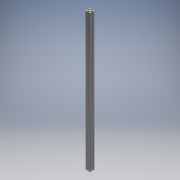
# Autodesk Inventor part: 4040_Alu
Saved by Autodesk Inventor 2019 (Build 230136000, 136)
## iProperties
Created: 2018-02-07
Part Number: 4040_Alu
Material: Aluminum 6061
Document SubType Name: Modeling
Designer: thijs
Density: 2.7 g/cm^3
Appearance: Aluminum - Polished
Author: thijs
Autodesk Inventor part; units mm, degrees
ref_plane "YZ Plane" through (0, 0, 0) normal (1, 0, 0) x (0, 1, 0)
ref_plane "XZ Plane" through (0, 0, 0) normal (0, 1, 0) x (-1, 0, 0)
ref_plane "XY Plane" through (0, 0, 0) normal (0, 0, 1) x (1, 0, 0)
sketch "Sketch1" plane through (0, 0, 0) normal (0, 0, 1) x (1, 0, 0)
  line L0 (7.425, -7.425) -> (-7.425, -7.425)
  line L1 (-7.425, -7.425) -> (-7.425, 7.425)
  line L2 (-7.425, 7.425) -> (7.425, 7.425)
  line L3 (7.425, 7.425) -> (7.425, -7.425)
  line L4 (7.425, -7.425) -> (-7.425, 7.425) construction
  line L5 (-7.425, -7.425) -> (7.425, 7.425) construction
  line L6 (20, -20) -> (-20, -20)
  line L7 (-20, -20) -> (-20, 20)
  line L8 (-20, 20) -> (20, 20)
  line L9 (20, 20) -> (20, -20)
  line L10 (20, -20) -> (-20, 20) construction
  line L11 (-20, -20) -> (20, 20) construction
  line L12 (-16.1503, -19.205) -> (19.205, 16.1503)
  line L13 (19.205, 16.1503) -> (16.1503, 19.205)
  line L14 (16.1503, 19.205) -> (-19.205, -16.1503)
  line L15 (-19.205, -16.1503) -> (-16.1503, -19.205)
  line L16 (-16.1503, -19.205) -> (16.1503, 19.205) construction
  line L17 (19.205, 16.1503) -> (-19.205, -16.1503) construction
  line L18 (16.1503, -19.205) -> (-19.205, 16.1503)
  line L19 (-19.205, 16.1503) -> (-16.1503, 19.205)
  line L20 (-16.1503, 19.205) -> (19.205, -16.1503)
  line L21 (19.205, -16.1503) -> (16.1503, -19.205)
  line L22 (16.1503, -19.205) -> (-16.1503, 19.205) construction
  line L23 (-19.205, 16.1503) -> (19.205, -16.1503) construction
  line L24 (-20, 20) -> (-15.68, 20)
  line L25 (-15.68, 20) -> (-15.68, 4.065)
  line L26 (-15.68, 4.065) -> (-20, 4.065)
  line L27 (-20, 4.065) -> (-20, 20)
  line L28 (-20, -20) -> (-15.68, -20)
  line L29 (-15.68, -20) -> (-15.68, -4.065)
  line L30 (-15.68, -4.065) -> (-20, -4.065)
  line L31 (-20, -4.065) -> (-20, -20)
  line L32 (-20, 20) -> (-4.32, 20)
  line L33 (-4.32, 20) -> (-4.32, 15.68)
  line L34 (-4.32, 15.68) -> (-20, 15.68)
  line L35 (-20, 15.68) -> (-20, 20)
  line L36 (20, 20) -> (3.81, 20)
  line L37 (3.81, 20) -> (3.81, 15.68)
  line L38 (3.81, 15.68) -> (20, 15.68)
  line L39 (20, 15.68) -> (20, 20)
  line L40 (20, -20) -> (15.68, -20)
  line L41 (15.68, -20) -> (15.68, -4.32)
  line L42 (15.68, -4.32) -> (20, -4.32)
  line L43 (20, -4.32) -> (20, -20)
  line L44 (20, -20) -> (4.065, -20)
  line L45 (4.065, -20) -> (4.065, -15.68)
  line L46 (4.065, -15.68) -> (20, -15.68)
  line L47 (20, -15.68) -> (20, -20)
  line L48 (-20, -20) -> (-4.065, -20)
  line L49 (-4.065, -20) -> (-4.065, -15.68)
  line L50 (-4.065, -15.68) -> (-20, -15.68)
  line L51 (-20, -15.68) -> (-20, -20)
  line L52 (20, 20) -> (15.68, 20)
  line L53 (15.68, 20) -> (15.68, 3.81)
  line L54 (15.68, 3.81) -> (20, 3.81)
  line L55 (20, 3.81) -> (20, 20)
  point P0 (0, 0)
  dimension "d0" = 14.85
  dimension "d1" = 14.85
  dimension "d2" = 40
  dimension "d3" = 40
  dimension "d4" = 4.32
  dimension "d5" = 4.32
  dimension "d6" = 50
  dimension "d7" = 50
  dimension "d8" = 4.32
  dimension "d10" = 4.32
  dimension "d11" = 8.13
  dimension "d12" = 4.065
  dimension "d15" = 4.32
  dimension "d16" = 4.32
  dimension "d17" = 4.32
  dimension "d18" = 4.32
  dimension "d19" = 8.13
  dimension "d20" = 8.13
  dimension "d21" = 4.065
  dimension "d22" = 4.32
  dimension "d23" = 4.32
  dimension "d24" = 4.32
  dimension "d25" = 8.13
  dimension "d26" = 4.32
  dimension "d28" = 8.255
  constraints: 112 end point, 26 parallel, 12 perpendicular, 10 horizontal, 8 midpoint, 1 point on line
  measures "d0" distance of L1.end L2.end
  measures "d1" distance of L0.end L1.end
  measures "d2" distance of L7.end L8.end
  measures "d3" distance of L6.end L7.end
  measures "d4" distance of L13.end L12.end
  measures "d5" distance of L18.end L19.end
  measures "d6" distance of L12.start L12.end
  measures "d7" distance of L19.end L20.end
  measures "d8" distance of L25.end L26.end
  measures "d10" distance of L30.end L29.end
  measures "d11" distance between parallel lines of L30 L26
  measures "d12" distance from line of point (0, 0) L26
  measures "d15" distance of L48.end L49.end
  measures "d16" distance of L44.end L45.end
  measures "d17" distance of L36.end L37.end
  measures "d18" distance of L32.end L33.end
  measures "d19" distance between parallel lines of L37 L33
  measures "d20" distance between parallel lines of L49 L45
  measures "d21" distance from line of point (0, 0) L49
  measures "d22" distance from line of point (0, 0) L33
  measures "d23" distance from line of L42 point (0, 0)
  measures "d24" distance of L41.end L42.end
  measures "d25" distance between parallel lines of L42 L54
  measures "d26" distance of L53.end L54.end
  measures "d28" distance between parallel lines of L29 L1
extrude "Extrusion1" add sketch "Sketch1" along normal blind 1200 contours L3 L20 L41 L46 L18 L0 | L0 L18 L12 L20 L3 | L0 L12 L18 | L20 L12 L3 | L12 L50 L29 L14 L1 L0 | L0 L1 L14 L18 L12 | L46 L41 L18 | L18 L41 L6 L45 L46 | L18 L14 L20 L12 | L12 L20 L14 L2 L3 | L3 L2 L14 L38 L53 L12 | L41 L42 L9 L46 L20 | L20 L46 L41 | L50 L49 L6 L29 L12 | L12 L29 L50 | L41 L46 L20 L21 L18 | L18 L21 L20 L46 L9 L6 L41 | L18 L1 L2 L20 L14 | L14 L1 L18 | L53 L38 L12 | L12 L38 L9 L54 L53 | L20 L2 L14 | L29 L6 L7 L50 L14 L15 L12 | L12 L15 L14 L50 L29 | L50 L14 L29 | L18 L25 L34 L20 L2 L1 | L38 L53 L14 L13 L12 | L12 L13 L14 L53 L8 L9 L38 | L38 L14 L53 | L14 L50 L7 L30 L29 | L25 L26 L7 L34 L18 | L18 L34 L25 | L38 L37 L8 L53 L14 | L34 L25 L20 | L20 L25 L8 L33 L34 | L34 L7 L8 L25 L20 L19 L18 | L18 L19 L20 L25 L34
fillet "Fillet1" radius 2 19 edges at (12.6253, 15.68, 600) (15.68, 12.6253, 600) (20, 20, 600) (20, -20, 600) (7.425, -4.3703, 600) (7.425, 4.3703, 600) (15.68, -12.6253, 600) (12.6253, -15.68, 600) (-12.6253, -15.68, 600) (-15.68, -12.6253, 600) (-20, -20, 600) (-7.425, -4.3703, 600) (-4.3703, -7.425, 600) (-7.425, 4.3703, 600) (-4.3703, 7.425, 600) (4.3703, 7.425, 600) (-12.6253, 15.68, 600) (-20, 20, 600) (-15.68, 12.6253, 600)
fillet "Fillet1" radius 1.5 16 edges at (-15.68, 4.065, 600) (-20, 4.065, 600) (-4.32, 20, 600) (-4.32, 15.68, 600) (3.81, 15.68, 600) (3.81, 20, 600) (20, 3.81, 600) (15.68, 3.81, 600) (15.68, -4.32, 600) (20, -4.32, 600) (4.065, -20, 600) (4.065, -15.68, 600) (-4.065, -20, 600) (-4.065, -15.68, 600) (-15.68, -4.065, 600) (-20, -4.065, 600)
sketch "Sketch2" plane through (0, 0, 1200) normal (0, 0, 1) x (1, 0, 0)
  circle A0 centre (0, 0) radius 3.405
  dimension "d30" = 6.81
  constraints: 1 centre point, 1 coincident
  measures "d30" diameter of A0
extrude "Extrusion2" cut sketch "Sketch2" against normal through all
sketch "Skizze3" plane through (0, 0, 1200) normal (0, 0, 1) x (1, 0, 0)
  point P0 (0, 0)
equation "\"d1\" = d0"
equation "\"d7\" = d6"
equation "\"d12\" = 0.5 * d11"
equation "\"d15\" = d8"
equation "\"d17\" = d8"
equation "\"d18\" = d8"
equation "\"d19\" = d11"
equation "\"d20\" = d19"
equation "\"d21\" = d12"
equation "\"d22\" = d8"
equation "\"d23\" = d8"
equation "\"d24\" = d8"
equation "\"d25\" = d11"
equation "\"d26\" = d8"
body "Solid1"
